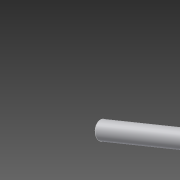
# Autodesk Inventor part: Stift01
Saved by Autodesk Inventor 2013 (Build 170138000, 138)
## iProperties
Created: 2006-10-06
Part Number: Stift01
Document SubType Name: Modeling
Designer: acad
Manufacturer: Standard
Standards Organization: Custom
Material: Allgemein
Density: 1 g/cm^3
Author: acad
Autodesk Inventor part; units mm, degrees
ref_plane "YZ Plane" through (0, 0, 0) normal (1, 0, 0) x (0, 1, 0)
ref_plane "XZ Plane" through (0, 0, 0) normal (0, 1, 0) x (-1, 0, 0)
ref_plane "XY Plane" through (0, 0, 0) normal (0, 0, 1) x (1, 0, 0)
sketch "Skizze1" plane through (0, 0, 0) normal (0, 0, 1) x (1, 0, 0)
  circle A0 centre (0, 0) radius 0.75
  dimension "d0" = 1.5
  dimension "d0" = 1.5
  constraints: 1 centre point
  measures "d0" diameter of A0
extrude "Extrusion1" add sketch "Skizze1" along normal blind 3.9
